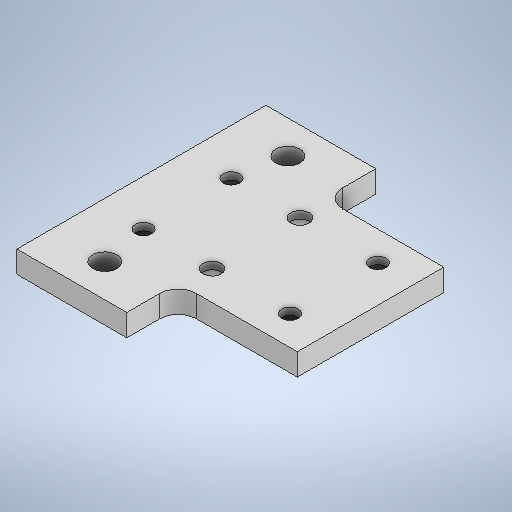
# Autodesk Inventor part: TS_Halterung_Fuehrungszylinder_int
Saved by Autodesk Inventor 2025.2 (Build 292293000, 293)
## iProperties
Created: 2025-06-19
Part Number: TS_Halterung_Fuehrungszylinder_int
Material: Generisch
Document SubType Name: Modeling
Designer: tino
Density: 1 g/cm^3
Appearance: Vorgabe
Author: tino
Autodesk Inventor part; units mm, degrees
ref_plane "YZ Plane" through (0, 0, 0) normal (1, 0, 0) x (0, 1, 0)
ref_plane "XZ Plane" through (0, 0, 0) normal (0, 1, 0) x (-1, 0, 0)
ref_plane "XY Plane" through (0, 0, 0) normal (0, 0, 1) x (1, 0, 0)
sketch "Skizze1" plane through (0, 0, 0) normal (0, 0, 1) x (1, 0, 0)
  line L0 (-31.2875, 34) -> (31.2875, 34)
  line L1 (31.2875, 34) -> (31.2875, -34)
  line L2 (31.2875, -34) -> (-31.2875, -34)
  line L3 (-31.2875, -34) -> (-31.2875, 34)
  point P0 (0, 0)
  dimension "d0" = 62.575
  dimension "d1" = 68
  dimension "d40" = 31.2875
  dimension "d41" = 34
  constraints: 8 end point, 2 parallel, 1 horizontal, 1 perpendicular
  measures "d0" distance of L0.start L0.end
  measures "d1" distance of L0.end L1.end
  measures "d40" distance from line of L3 point (0, 0)
  measures "d41" distance from line of L0 point (0, 0)
extrude "Extrusion1" add sketch "Skizze1" along normal blind 6
sketch "Skizze2" plane through (0, 0, 0) normal (0, 0, -1) x (-1, 0, 0)
  line L0 (31.2875, 34) -> (31.2875, -34) projected
  point P0 (18.7125, -12)
  point P1 (-21.2875, -12)
  point P2 (0, 0)
  point P3 (-21.2875, 12)
  point P4 (18.7125, 12)
  point P5 (-21.2875, -12)
  dimension "d9" = 40
  dimension "d10" = 12.575
  dimension "d20" = 24
  dimension "d21" = 12
  constraints: 2 horizontal alignment, 2 vertical alignment, 1 coincident
  measures "d9" distance of point (-21.288, -12) point (18.712, -12)
  measures "d10" distance from line of L0 point (18.712, -12)
  measures "d20" distance of point (-21.288, 12) point (-21.288, -12)
  measures "d21" vertical distance of point (0, 0) point (-21.288, 12)
hole "Bohrung1" at (-18.7125, -12, 0) at (21.2875, -12, 0) at (21.2875, 12, 0) at (-18.7125, 12, 0) direction (0, 0, 1) diameter 4.5 end through all counterbore diameter 8 counterbore depth 4 clearance for "Innensechskantkopfschraube" size "M4" standard "ANSI Metrisches M Profil"
sketch "Skizze3" plane through (0, 0, 6) normal (0, 0, 1) x (1, 0, 0)
  circle A0 centre (21.2875, -12) radius 2.25 projected
  circle A1 centre (-18.7125, -12) radius 2.25 projected
  circle A2 centre (-18.7125, 12) radius 2.25 projected
  circle A3 centre (21.2875, 12) radius 2.25 projected
  point P0 (0, 0)
  point P1 (0, -12)
  point P2 (0, 12)
  constraints: 2 horizontal alignment, 2 vertical alignment
hole "Bohrung2" at (0, -12, 6) at (0, 12, 6) direction (0, 0, -1) diameter 5 depth 2
sketch "Skizze4" plane through (0, 0, 6) normal (0, 0, 1) x (1, 0, 0)
  line L0 (-31.2875, -34) -> (31.2875, -34) projected
  line L1 (31.2875, 34) -> (-31.2875, 34) projected
  line L2 (-31.2875, 34) -> (-31.2875, -34) projected
  point P0 (0, 0)
  point P1 (-16.2875, -25)
  point P2 (-16.2875, 25)
  dimension "d29" = 9
  dimension "d30" = 9
  dimension "d31" = 15
  constraints: 1 vertical alignment
  measures "d29" distance from line of L0 point (-16.287, -25)
  measures "d30" distance from line of L1 point (-16.287, 25)
  measures "d31" distance from line of L2 point (-16.287, -25)
hole "Bohrung3" at (-16.2875, -25, 6) at (-16.2875, 25, 6) direction (0, 0, -1) diameter 6.6 end through all clearance for "Innensechskantkopfschraube" size "M6" standard "ANSI Metrisches M Profil"
sketch "Skizze5" plane through (0, 0, 6) normal (0, 0, 1) x (1, 0, 0)
  line L0 (-31.2875, -34) -> (31.2875, -34) projected
  line L1 (31.2875, -34) -> (31.2875, 34) projected
  line L2 (-1.2875, -34) -> (31.2875, -34)
  line L3 (31.2875, -34) -> (31.2875, -20)
  line L4 (31.2875, -20) -> (3.7125, -20)
  line L5 (-1.2875, -25) -> (-1.2875, -34)
  line L6 (-1.2875, 34) -> (31.2875, 34)
  line L7 (31.2875, 34) -> (31.2875, 20)
  line L8 (31.2875, 20) -> (3.7125, 20)
  line L9 (-1.2875, 25) -> (-1.2875, 34)
  line L10 (-31.2875, 34) -> (-31.2875, -34) projected
  line L11 (31.2875, 34) -> (-31.2875, 34) projected
  arc A0 (3.7125, -20) -> (-1.2875, -25) centre (3.7125, -25) ccw
  arc A1 (-1.2875, 25) -> (3.7125, 20) centre (3.7125, 25) ccw
  point P0 (0, 0)
  point P1 (-1.2875, -29.5)
  dimension "d42" = 40
  dimension "d43" = 20
  dimension "d44" = 30
  dimension "d45" = 30
  dimension "d46" = 5
  constraints: 16 end point, 4 parallel, 4 point on circle, 4 point on line, 4 tangent, 2 centre point, 2 horizontal, 2 perpendicular, 1 collinear, 1 equal radius, 1 midpoint
  measures "d42" distance between parallel lines of L8 L4
  measures "d43" distance from line of L4 point (0, 0)
  measures "d44" distance from line of L10 point (-1.287, -29.5)
  measures "d45" distance between parallel lines of L10 L9
  measures "d46" radius of A0
extrude "Extrusion2" cut sketch "Skizze5" against normal through all contours L5 A0 L4 L1 L0 | L6 L1 L8 A1 L9
equation "\"d40\" = 0.5 * d0"
equation "\"d41\" = 0.5 * d1"
